Autodesk Fusion 360 part; units mm, degrees
(part 2 of 2)
sketch "Schizzo10" plane through (0, 0, 82.5) normal (0, 0, 1) x (-1, 0, 0)
  line L0 (-215.0609, -225.7386) -> (-305.0609, -225.7386)
  line L1 (-305.0609, -225.7386) -> (-305.0609, -254.7386)
  line L2 (-305.0609, -254.7386) -> (-215.0609, -254.7386)
  line L3 (-217.0609, -240.2386) -> (-305.0609, -240.2386) construction
  line L4 (-260.0609, -254.7386) -> (-260.0609, -225.7386) construction
  line L5 (-215.0609, -254.7386) -> (-305.0609, -254.7386)
  line L6 (-305.0609, -254.7386) -> (-305.0609, -225.7386)
  line L7 (-305.0609, -225.7386) -> (-215.0609, -225.7386)
  line L8 (-215.0609, -225.7386) -> (-215.0609, -254.7386)
  line L9 (-274.0609, -262) -> (-274.0609, -222) construction
  line L10 (-303.0609, -237) -> (-303.0609, -262) construction
  arc A0 (-289.5609, -226.7386) -> (-289.5609, -253.7386) centre (-289.5609, -240.2386) ccw construction
  line L11 (-217.0609, -227.7386) -> (-303.0609, -227.7386)
  line L12 (-303.0609, -227.7386) -> (-303.0609, -252.7386)
  line L13 (-303.0609, -252.7386) -> (-217.0609, -252.7386)
  line L14 (-217.0609, -252.7386) -> (-217.0609, -227.7386)
  line L15 (-228.8609, -252.7386) -> (-243.2609, -252.7386)
  line L16 (-243.2609, -252.7386) -> (-243.2609, -247.5386)
  line L17 (-243.2609, -247.5386) -> (-228.8609, -247.5386)
  line L18 (-228.8609, -247.5386) -> (-228.8609, -252.7386)
  line L19 (-228.8609, -232.9386) -> (-228.8609, -227.7386)
  line L20 (-243.2609, -227.7386) -> (-243.2609, -232.9386)
  line L21 (-243.2609, -232.9386) -> (-228.8609, -232.9386)
  line L22 (-215.0609, -254.7386) -> (-215.0609, -225.7386)
  line L23 (-223.0609, -247.5386) -> (-243.2609, -247.5386)
  line L24 (-243.2609, -247.5386) -> (-243.2609, -244.3386)
  line L25 (-243.2609, -244.3386) -> (-223.0609, -244.3386)
  line L26 (-223.0609, -244.3386) -> (-223.0609, -247.5386)
  line L27 (-223.0609, -236.1386) -> (-223.0609, -232.9386)
  line L28 (-223.0609, -232.9386) -> (-243.2609, -232.9386)
  line L29 (-243.2609, -236.1386) -> (-223.0609, -236.1386)
  line L30 (-243.2609, -232.9386) -> (-243.2609, -236.1386)
  line L31 (-299.0609, -230.7386) -> (-303.0609, -230.7386)
  line L32 (-303.0609, -230.7386) -> (-303.0609, -227.7386)
  line L33 (-303.0609, -227.7386) -> (-299.0609, -227.7386)
  line L34 (-299.0609, -227.7386) -> (-299.0609, -230.7386)
  line L35 (-303.0609, -227.7386) -> (-300.0609, -227.7386)
  line L36 (-300.0609, -227.7386) -> (-300.0609, -231.7386)
  line L37 (-300.0609, -231.7386) -> (-303.0609, -231.7386)
  line L38 (-303.0609, -231.7386) -> (-303.0609, -227.7386)
  line L39 (-299.0609, -249.7386) -> (-303.0609, -249.7386)
  line L40 (-300.0609, -252.7386) -> (-300.0609, -248.7386)
  line L41 (-300.0609, -248.7386) -> (-303.0609, -248.7386)
  line L42 (-303.0609, -249.7386) -> (-303.0609, -252.7386)
  line L43 (-303.0609, -248.7386) -> (-303.0609, -252.7386)
  line L44 (-299.0609, -252.7386) -> (-299.0609, -249.7386)
  line L45 (-303.0609, -252.7386) -> (-300.0609, -252.7386)
  point P0 (-260.0609, -240.2386)
  point P1 (-274.0609, -240.2386)
  dimension "d190" = 29
  dimension "d207" = 2
  dimension "d208" = 2
  dimension "d209" = 2
  dimension "d210" = 2
  dimension "d215" = 14.4
  dimension "d216" = 5.2
  dimension "d217" = 13.8
  dimension "d387" = 20.2
  dimension "d388" = 3.2
  dimension "d425" = 4
  dimension "d426" = 3
  dimension "d427" = 3
  dimension "d428" = 4
  constraint midpoint L1 L3.end
  constraint midpoint L2 L4.start
  constraint midpoint L0 L4.end
  constraint midpoint L4 P0
  constraint horizontal L5
  constraint vertical L6
  constraint horizontal L7
  constraint vertical L8
  constraint coincident L2.end L5.start
  constraint coincident L0.end L1.start
  constraint perpendicular L0 L9
  constraint perpendicular L2 L10
  constraint tangent L10 A0
  constraint coincident L9 P1
  constraint coincident L3 P1
  constraint horizontal L11
  constraint vertical L12
  constraint horizontal L13
  constraint vertical L14
  constraint horizontal L15
  constraint vertical L16
  constraint horizontal L17
  constraint vertical L18
  constraint collinear L13 L15
  constraint symmetric L3 L15.start L19.end
  constraint symmetric L3 L15.end L20.start
  constraint symmetric L3 L16.end L20.end
  constraint symmetric L3 L17.end L19.start
  constraint horizontal L23
  constraint vertical L24
  constraint horizontal L25
  constraint vertical L26
  constraint coincident L16.end L17.start
  constraint symmetric L3 L23.start L27.end
  constraint symmetric L3 L24.end L29.start
  constraint symmetric L3 L25.end L27.start
  constraint horizontal L31
  constraint vertical L32
  constraint horizontal L33
  constraint vertical L34
  constraint horizontal L35
  constraint vertical L36
  constraint horizontal L37
  constraint vertical L38
  constraint coincident L11.end L12.start
  constraint symmetric L3 L31.start L39.start
  constraint symmetric L3 L31.end L39.end
  constraint symmetric L3 L11.end L12.end
  constraint symmetric L3 L33.end L44.start
  constraint symmetric L3 L35.end L40.start
  constraint symmetric L3 L36.end L40.end
  constraint symmetric L3 L37.end L41.end
  measures "d190" distance of L9 L10
  measures "d207" distance of L6 L12
  measures "d208" distance of L5 L13
  measures "d209" distance of L7 L11
  measures "d210" distance of L8 L14
  measures "d215" distance of L15.start L15.end
  measures "d216" distance of L15 L17
  measures "d217" distance of L8 L18
  measures "d387" distance of L23.start L16.end
  measures "d388" distance of L23.start L25.end
  measures "d425" distance of L31.start L31.end
  measures "d426" distance of L31.start L33.end
  measures "d427" distance of L11.end L35.end
  measures "d428" distance of L33 L37
extrude "Estrusione45" add sketch "Schizzo1" along normal blind 5 separate body contours L94 L95 L96 L97 L100 L101 L102 L103 L104 L105 | L94 L99 L100 L101 L102 | L96 L103 L104 L105 L106 makes body 13
extrude "Estrusione44" add sketch "Schizzo1" along normal blind 56 contours L90 L91 L92 L93 bodies 13
extrude "Estrusione49" add sketch "Schizzo1" along normal blind 70 contours L94 L99 L100 L101 L102 | L96 L103 L104 L105 L106 bodies 13
sketch "Blocco Coperchio 1" plane through (0, 223, 0) normal (0, -1, 0) x (1, 0, 0)
  line L0 (110.9231, 56) -> (124.9231, 56)
  line L1 (124.9231, 56) -> (124.9231, 70)
  line L2 (124.9231, 70) -> (110.9231, 70)
  line L3 (110.9231, 70) -> (110.9231, 56)
  circle A0 centre (117.9231, 64) radius 3
  line L4 (138.9231, 0) -> (138.9231, 56)
  line L5 (48.9231, 56) -> (138.9231, 56)
  circle A1 centre (117.9231, 64) radius 1.5
  dimension "d351" = 6
  dimension "d369" = 21
  dimension "d370" = 8
  dimension "d371" = 3
  constraint concentric A0 A1
  measures "d351" diameter of A0
  measures "d369" distance of A0.centre L4
  measures "d370" distance of A0.centre L5
  measures "d371" diameter of A1
extrude "Estrusione73" cut sketch "Blocco Coperchio 1" against normal blind 1 contours A0 | A1 bodies 13
extrude "Estrusione75" cut sketch "Blocco Coperchio 1" against normal blind 30 contours A1 bodies 13
sketch "Schizzo21" plane through (0, 248, 0) normal (0, 1, 0) x (-1, 0, 0)
  circle A0 centre (-117.9231, 64) radius 1.5
  line L0 (-124.9231, 56) -> (-110.9231, 56)
  line L1 (-110.9231, 56) -> (-110.9231, 70)
  line L2 (-110.9231, 70) -> (-124.9231, 70)
  line L3 (-124.9231, 70) -> (-124.9231, 56)
  line L4 (-117.9231, 64) -> (-110.9231, 63) construction
  line L5 (-117.9231, 64) -> (-117.9231, 70) construction
  circle A1 centre (-117.9231, 64) radius 3
  dimension "d374" = 6
  constraint coincident A0.centre L4.start
  constraint midpoint L1 L4.end
  constraint midpoint L2 L5.end
  measures "d374" diameter of A1
extrude "Estrusione76" cut sketch "Schizzo21" against normal blind 1 contours A1 bodies 13
extrude "Estrusione48" cut sketch "Schizzo10" against normal blind 25 from surface at 3 contours L11 L19 L20 L21 L28 | L13 L15 L16 L17 L18 L23 bodies 12
sketch "Schizzo13" plane through (0, 225.7386, 0) normal (0, -1, 0) x (1, 0, 0)
  circle A0 centre (273.0609, 41.75) radius 11
  line L0 (305.0609, 0) -> (305.0609, 82.5)
  line L1 (236.0609, 83.5) -> (236.0609, 0) construction
  line L2 (215.0609, 74.5) -> (305.0609, 74.5) construction
  circle A1 centre (236.0609, 74.5) radius 1.4
  circle A2 centre (236.0609, 74.5) radius 3
  line L3 (305.0609, 82.5) -> (215.0609, 82.5)
  line L4 (215.0609, 82.5) -> (215.0609, 0)
  line L5 (215.0609, 0) -> (305.0609, 0)
  dimension "d252" = 2.8
  dimension "d253" = 6
  dimension "d367" = 8
  dimension "d368" = 21
  constraint coincident L0 L2.end
  constraint coincident L1 A1.centre
  constraint coincident L2 A1.centre
  constraint concentric A1 A2
  measures "d252" diameter of A1
  measures "d253" diameter of A2
  measures "d367" distance of L2 L3
  measures "d368" distance of L1 L4
extrude "Estrusione54" cut sketch "Schizzo13" against normal blind 30 contours A1 bodies 12
extrude "Estrusione55" cut sketch "Schizzo13" against normal blind 3.5 contours A2 bodies 12
sketch "Schizzo14" plane through (0, 254.7386, 0) normal (0, 1, 0) x (-1, 0, 0)
  circle A0 centre (-236.0609, 74.5) radius 1.4
  line L0 (-305.0609, 82.5) -> (-305.0609, 0)
  line L1 (-236.0609, 74.5) -> (-226.9999, 74.5027) construction
  line L2 (-236.0609, 74.5) -> (-236.06, 71.5) construction
  circle A1 centre (-236.0609, 74.5) radius 3
  line L3 (-215.0609, 0) -> (-215.0609, 82.5)
  line L4 (-215.0609, 82.5) -> (-305.0609, 82.5)
  line L5 (-305.0609, 0) -> (-215.0609, 0)
  dimension "d258" = 6
  constraint coincident A0.centre L1.start
  constraint perpendicular L1 L2
  measures "d258" diameter of A1
extrude "Estrusione56" cut sketch "Schizzo14" against normal blind 3.5 contours A1 bodies 12
sketch "Schizzo18" plane through (0, 221, 0) normal (0, -1, 0) x (1, 0, 0)
  line L0 (48.9231, 0) -> (138.9231, 0)
  line L1 (138.9231, 0) -> (138.9231, 56)
  line L2 (138.9231, 56) -> (48.9231, 56)
  line L3 (48.9231, 56) -> (48.9231, 0)
  line L4 (55.9231, 49) -> (64.4231, 49)
  line L5 (64.4231, 49) -> (64.4231, 35)
  line L6 (64.4231, 35) -> (55.9231, 35)
  line L7 (55.9231, 35) -> (55.9231, 49)
  line L8 (55.9231, 16) -> (81.9231, 16)
  line L9 (81.9231, 16) -> (81.9231, 0)
  line L10 (81.9231, 0) -> (55.9231, 0)
  line L11 (55.9231, 0) -> (55.9231, 16)
  line L12 (0, 0) -> (100, 0) construction
  line L13 (68.9231, 16) -> (68.9231, 0) construction
  line L14 (55.9231, 8) -> (81.9231, 8) construction
  line L15 (71.4231, 5.5) -> (66.4231, 5.5)
  line L16 (66.4231, 5.5) -> (66.4231, 10.5)
  line L17 (66.4231, 10.5) -> (71.4231, 10.5)
  line L18 (71.4231, 10.5) -> (71.4231, 5.5)
  line L19 (71.4231, 5.5) -> (66.4231, 10.5) construction
  line L20 (66.4231, 5.5) -> (71.4231, 10.5) construction
  line L21 (55.9231, 12.6) -> (81.9231, 12.6) construction
  line L22 (63.4231, 16) -> (63.4231, 0) construction
  circle A0 centre (63.4231, 12.6) radius 1.4
  circle A1 centre (74.4231, 12.6) radius 1.4
  circle A2 centre (63.4231, 3.4) radius 1.4
  circle A3 centre (74.4231, 3.4) radius 1.4
  line L23 (71.4231, 5.5) -> (71.4231, 10.5)
  line L24 (71.4231, 10.5) -> (71.4231, 16) construction
  line L25 (66.4231, 16) -> (71.4231, 16)
  line L26 (71.4231, 16) -> (71.4231, 10.5)
  line L27 (71.4231, 10.5) -> (66.4231, 10.5)
  line L28 (66.4231, 10.5) -> (66.4231, 16)
  point P0 (68.9231, 8)
  dimension "d325" = 8.5
  dimension "d326" = 14
  dimension "d328" = 7
  dimension "d332" = 16
  dimension "d334" = 7
  dimension "d335" = 26
  dimension "d336" = 5
  dimension "d337" = 5
  dimension "d338" = 3.4
  dimension "d339" = 7.5
  dimension "d340" = 2.8
  constraint horizontal L4
  constraint vertical L5
  constraint horizontal L6
  constraint vertical L7
  constraint horizontal L8
  constraint vertical L9
  constraint horizontal L10
  constraint vertical L11
  constraint collinear L10 L12
  constraint collinear L7 L11
  constraint midpoint L8 L13.start
  constraint midpoint L10 L13.end
  constraint midpoint L11 L14.start
  constraint midpoint L9 L14.end
  constraint horizontal L15
  constraint perpendicular L15 L16
  constraint parallel L15 L17
  constraint parallel L16 L18
  constraint coincident L19 P0
  constraint coincident L20 P0
  constraint midpoint L13 P0
  constraint coincident L11 L21.start
  constraint coincident L9 L21.end
  constraint perpendicular L9 L21
  constraint coincident L8 L22.start
  constraint coincident L10 L22.end
  constraint coincident L22 A0.centre
  constraint coincident L21 A0.centre
  constraint symmetric L13 A0 A1
  constraint symmetric L14 A0 A2
  constraint symmetric L14 A1 A3
  constraint vertical L23
  constraint coincident L8 L24.end
  constraint perpendicular L8 L24
  constraint horizontal L25
  constraint vertical L26
  constraint horizontal L27
  constraint vertical L28
  constraint coincident L16.end L17.start
  constraint coincident L24.end L25.end
  measures "d325" distance of L4.start L4.end
  measures "d326" distance of L4.start L6.end
  measures "d328" distance of L2 L4
  measures "d332" distance of L8.start L10.end
  measures "d334" distance of L3 L11
  measures "d335" distance of L9 L11
  measures "d336" distance of L16.end L17.end
  measures "d337" distance of L15.end L16.end
  measures "d338" distance of L8 L21
  measures "d339" distance of L11 L22
  measures "d340" diameter of A0
extrude "Estrusione68" cut sketch "Schizzo18" against normal blind 5 contours L4 L5 L6 L7 bodies 13
extrude "Estrusione69" add sketch "Schizzo18" against normal blind 29 contours L0 L8 L9 L10 L11 L15 L16 L18 L23 L26 L28 | L8 L17 L25 L26 L27 L28 | L15 L16 L17 L18 L23 L27 bodies 13
extrude "Estrusione70" cut sketch "Schizzo18" against normal blind 20 contours A0 | A1 | A2 | A3 bodies 13
extrude "Estrusione94" cut sketch "Schizzo18" against normal blind 15 contours L15 L16 L17 L18 L23 L27 bodies 13
extrude "Estrusione95" cut sketch "Schizzo18" against normal blind 10 from surface at -5 contours L8 L17 L25 L26 L27 L28 bodies 13
extrude "Estrusione77" add sketch "Schizzo1" against normal blind 4 separate body contours L127 L141 L143 L176 L181 | L124 L137 L139 L173 L178 makes body 14 at (421.8629, 245.2895, -1.3333) makes body 15 at (415.8629, 230.6895, -1.3333)
extrude "Estrusione78" add sketch "Schizzo1" along normal blind 3 contours L86 L87 L88 L89 L123 L125 L126 L128 L137 L138 L139 L140 L141 L142 L143 L144 L150 L153 L154 L157 L158 L159 L160 L161 L164 L166 L167 L168 L170 L171 L174 L175 L177 L179 L180 | L127 L141 L143 L176 L181 | L86 L150 L152 L153 L157 | L127 L141 L143 L144 L176 | L141 L142 L143 L181 | L86 L87 L150 L151 L152 L155 L156 L157 | L87 L150 L154 L155 L157 | L124 L137 L139 L173 L178 | L88 L158 L159 L161 L162 | L124 L137 L138 L139 L172 L173 L174 L175 | L137 L139 L140 L177 L178 L179 L180 | L87 L88 L159 L161 L162 L163 | L87 L159 L160 L161 L163 bodies 14 15
extrude "Estrusione79" cut sketch "Schizzo10" against normal blind 5 contours L21 L27 L28 L29 L30 | L17 L23 L24 L25 L26 bodies 12
extrude "Estrusione80" add sketch "Schizzo1" along normal blind 20 separate body contours L145 L148 A34 | L145 L146 A34 | A34 | L146 L147 L148 A34 makes body 16
sketch "Schizzo22" plane through (0, 0, 0) normal (0, -1, 0) x (1, 0, 0)
  line L0 (380, 0) -> (396, 0)
  line L1 (396, 0) -> (396, 20)
  line L2 (396, 20) -> (380, 20)
  line L3 (380, 20) -> (380, 0)
  line L4 (388, 20) -> (388, 0) construction
  line L5 (380, 10) -> (396, 10) construction
  line L6 (380, 11.5) -> (396, 11.5)
  line L7 (396, 11.5) -> (396, 8.5)
  line L8 (396, 8.5) -> (380, 8.5)
  line L9 (380, 8.5) -> (380, 11.5)
  line L10 (390.25, 4.5) -> (394.75, 4.5)
  line L11 (394.75, 4.5) -> (394.75, 1.5)
  line L12 (394.75, 1.5) -> (390.25, 1.5)
  line L13 (390.25, 1.5) -> (390.25, 4.5)
  line L14 (390.25, 4.5) -> (396, 4.5)
  line L15 (396, 4.5) -> (396, 1.5)
  line L16 (396, 1.5) -> (390.25, 1.5)
  line L17 (390.25, 1.5) -> (390.25, 4.5)
  dimension "d403" = 3
  dimension "d458" = 4.5
  dimension "d459" = 3
  dimension "d460" = 1.25
  dimension "d461" = 1.5
  constraint midpoint L2 L4.start
  constraint midpoint L0 L4.end
  constraint midpoint L3 L5.start
  constraint midpoint L1 L5.end
  constraint horizontal L6
  constraint vertical L7
  constraint horizontal L8
  constraint vertical L9
  constraint midpoint L5.end L7
  constraint midpoint L3 L9
  constraint horizontal L10
  constraint vertical L11
  constraint horizontal L12
  constraint vertical L13
  constraint horizontal L14
  constraint vertical L15
  constraint horizontal L16
  constraint vertical L17
  constraint coincident L1 L15.end
  measures "d403" distance of L6.start L8.end
  measures "d458" distance of L10.start L10.end
  measures "d459" distance of L10.start L12.end
  measures "d460" distance of L1 L11
  measures "d461" distance of L0 L12
extrude "Estrusione81" cut sketch "Schizzo22" against normal blind 16.5 contours L1 L3 L6 L7 L8 L9 bodies 16
extrude "Estrusione82" cut sketch "Schizzo1" along normal blind 20 contours L145 L148 A34 | L145 L146 A34 bodies 16
sketch "Schizzo23" plane through (396, 0, 0) normal (1, 0, 0) x (0, 1, 0)
  line L0 (8, 20) -> (8, 11.5)
  line L1 (8, 11.5) -> (16.5, 11.5)
  line L2 (16.5, 11.5) -> (16.5, 8.5)
  line L3 (16.5, 8.5) -> (8, 8.5)
  line L4 (8, 8.5) -> (8, 0)
  line L5 (8, 0) -> (140, 0)
  line L6 (140, 0) -> (140, 20)
  line L7 (140, 20) -> (8, 20)
  line L8 (140, 10) -> (16.5, 10) construction
  line L9 (47, 19) -> (139, 19)
  line L10 (139, 19) -> (139, 1)
  line L11 (139, 1) -> (47, 1)
  line L12 (47, 1) -> (47, 19)
  line L13 (47, 10) -> (139, 10) construction
  line L14 (0, 0) -> (140, 0) construction
  circle A0 centre (32, 10) radius 3.25
  circle A1 centre (32, 10) radius 5
  line L15 (47, 19) -> (60, 19)
  line L16 (60, 19) -> (60, 1)
  line L17 (60, 1) -> (47, 1)
  line L18 (47, 1) -> (47, 19)
  dimension "d408" = 92
  dimension "d409" = 1
  dimension "d410" = 1
  dimension "d437" = 6.5
  dimension "d439" = 15
  dimension "d448" = 10
  dimension "d455" = 13
  constraint midpoint L6 L8.start
  constraint perpendicular L6 L8
  constraint horizontal L9
  constraint vertical L10
  constraint horizontal L11
  constraint vertical L12
  constraint midpoint L12 L13.start
  constraint midpoint L10 L13.end
  constraint collinear L8 L13
  constraint concentric A0 A1
  constraint horizontal L15
  constraint vertical L16
  constraint horizontal L17
  constraint vertical L18
  constraint coincident L9.start L12.end
  constraint coincident L11.end L12.start
  measures "d408" distance of L9.start L9.end
  measures "d409" distance of L6 L10.end
  measures "d410" distance of L11 L14
  measures "d437" diameter of A0
  measures "d439" distance of L12 A0.centre
  measures "d448" diameter of A1
  measures "d455" distance of L9.start L15.end
extrude "Estrusione83" cut sketch "Schizzo23" against normal blind 6 contours L9 L11 L12 L15 L16 L17 L18 | L9 L10 L11 L16 bodies 16
extrude "Estrusione85" cut sketch "Schizzo10" against normal blind 10 contours L11 L31 L33 L34 L36 | L11 L12 L31 L32 L33 L35 L36 L38 | L13 L39 L40 L44 | L12 L31 L36 L37 L38 | L12 L13 L39 L40 L42 L43 L45 | L12 L39 L40 L41 L43 bodies 12
extrude "Estrusione86" add sketch "Schizzo1" against normal blind 4 contours L86 L150 L152 L153 L157 | L86 L87 L150 L151 L152 L155 L156 L157 | L87 L150 L154 L155 L157 | L88 L158 L159 L161 L162 | L87 L88 L159 L161 L162 L163 | L87 L159 L160 L161 L163 bodies 14
extrude "Estrusione87" cut sketch "Schizzo23" against normal blind 16 contours A0 bodies 16
extrude "Estrusione88" add sketch "Schizzo1" along normal blind 4 separate body contours A37 makes body 17
extrude "Estrusione89" cut sketch "Schizzo23" against normal blind 6 contours A1 bodies 16
sketch "Schizzo24" plane through (380, 0, 0) normal (-1, 0, 0) x (0, -1, 0)
  circle A0 centre (-32, 10) radius 3.25
  line L0 (-8, 11.5) -> (-8, 20)
  line L1 (-8, 20) -> (-140, 20)
  line L2 (-140, 20) -> (-140, 0)
  line L3 (-140, 0) -> (-8, 0)
  line L4 (-8, 0) -> (-8, 8.5)
  line L5 (-8, 8.5) -> (-16.5, 8.5)
  line L6 (-16.5, 8.5) -> (-16.5, 11.5)
  line L7 (-16.5, 11.5) -> (-8, 11.5)
  line L8 (-32, 10) -> (-32, 20) construction
  line L9 (-32, 10) -> (-16.5, 10) construction
  line L10 (-19.5, 5) -> (-44.5, 5)
  line L11 (-44.5, 5) -> (-44.5, 15)
  line L12 (-44.5, 15) -> (-19.5, 15)
  line L13 (-19.5, 15) -> (-19.5, 5)
  line L14 (-19.5, 5) -> (-44.5, 15) construction
  line L15 (-44.5, 5) -> (-19.5, 15) construction
  point P0 (-32, 10)
  dimension "d451" = 25
  dimension "d452" = 10
  constraint coincident P0 A0.centre
  constraint coincident L1 L8.end
  constraint perpendicular L1 L8
  constraint midpoint L6 L9.end
  constraint horizontal L10
  constraint perpendicular L10 L11
  constraint parallel L10 L12
  constraint parallel L11 L13
  constraint coincident L14 P0
  constraint coincident L15 P0
  measures "d451" distance of L11.end L12.end
  measures "d452" distance of L10.end L11.end
extrude "Estrusione90" cut sketch "Schizzo24" against normal blind 5 contours L10 L11 L12 L13 bodies 16
extrude "Estrusione91" cut sketch "Schizzo23" against normal blind 10 contours L9 L11 L12 L15 L16 L17 L18 bodies 16
extrude "Estrusione92" cut sketch "Schizzo22" against normal blind 50 contours L10 L11 L12 L13 L14 L16 L17 bodies 16
extrude "Estrusione93" cut sketch "Schizzo22" against normal blind 17 contours L1 L11 L14 L15 L16 | L10 L11 L12 L13 L14 L16 L17 bodies 16
equation "d35 = BeamLenght"
equation "d61 = -BeamRelief"
equation "d65 = -BeamRelief"
equation "BeamLenght = 140 mm"
equation "d105 = BeamLenght"
equation "d112 = -BeamRelief"
equation "d116 = -BeamRelief"
equation "d150 = 110 mm - 22 mm + 2 mm"
equation "d160 = d158 - 2 * 2 mm"
equation "d197 = d150"
equation "d198 = d158"
equation "d200 = d199"
equation "d201 = d199"
equation "d202 = d199"
equation "d203 = 50 mm + 6 mm"
equation "d215 = 14 mm + 0.4 mm"
equation "d216 = 5 mm + 0.2 mm"
equation "d217 = 14 mm - 0.2 mm"
equation "d224 = 56 mm + 14 mm"
equation "d283 = ( ( 8.5 - 3 ) / 2 ) * 1 mm"
equation "d284 = d283"
equation "d295 = -BeamCableRelief"
equation "BeamRelief = 16.5 mm" comment "Questo lo scarico da usare nella trave per permettere la rotazione del giunto"
equation "d298 = -BeamCableRelief"
equation "BeamCableRelief = 17 mm"
equation "d309 = -BeamCableRelief"
equation "d377 = d150"
equation "d379 = 2.00 mm + 0.2 mm"
equation "d380 = 2 mm + 0.2 mm"
equation "d387 = 20 mm + 0.2 mm"
equation "d392 = BeamLenght"
equation "d404 = -BeamRelief"
equation "d431 = d434"
equation "d432 = 3 mm - 0.2 mm"
equation "d433 = d432"
equation "d434 = 4 mm - 0.2 mm"
equation "d464 = -BeamCableRelief"
named bodies: "Giunto di Base", "Ginto2Assi", "Giunto Allungato", "Beam", "Giunto Corto", "Tappo", "Batteria", "Lampada", "Blocco Filetto", "RetroBatteria"
